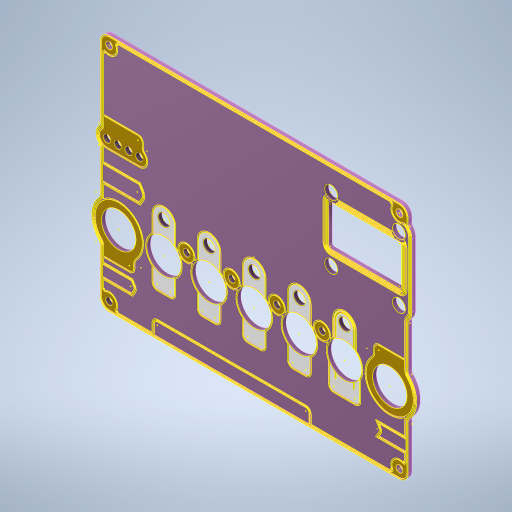
# Autodesk Inventor part: top_cover_template
Saved by Autodesk Inventor 2024 (Build 280153000, 153)
## iProperties
Created: 2023-11-30
Part Number: top_cover_template
Material: Generic
Document SubType Name: Modeling
Designer: Ishaan
Density: 1 g/cm^3
Appearance: Smooth - Purple
Author: Ishaan
Autodesk Inventor part; units mm, degrees
(part 1 of 4)
ref_plane "YZ Plane" through (0, 0, 0) normal (1, 0, 0) x (0, 1, 0)
ref_plane "XZ Plane" through (0, 0, 0) normal (0, 1, 0) x (-1, 0, 0)
ref_plane "XY Plane" through (0, 0, 0) normal (0, 0, 1) x (1, 0, 0)
sketch "Sketch1" plane through (0, 0, 0) normal (0, 0, 1) x (1, 0, 0)
  line L0 (71.5, -55.5) -> (-71.5, -55.5)
  line L1 (-71.5, -55.5) -> (-71.5, 55.5)
  line L2 (-71.5, 55.5) -> (71.5, 55.5)
  line L3 (71.5, 55.5) -> (71.5, -55.5)
  line L4 (71.5, -55.5) -> (-71.5, 55.5) construction
  line L5 (-71.5, -55.5) -> (71.5, 55.5) construction
  point P0 (0, 0)
  dimension "d0" = 143
  dimension "d1" = 111
  constraints: 12 end point, 2 midpoint, 2 parallel, 1 horizontal, 1 perpendicular
  measures "d0" distance of L1.end L2.end
  measures "d1" distance of L0.end L1.end
extrude "Extrusion1" add sketch "Sketch1" along normal blind 1.6
fillet "Fillet1" radius 4 4 edges at (71.5, 55.5, 0.8) (-71.5, 55.5, 0.8) (-71.5, -55.5, 0.8) (71.5, -55.5, 0.8)
sketch "Sketch2" plane through (0, 0, 1.6) normal (0, 0, 1) x (1, 0, 0)
  arc A0 (67.5, -55.5) -> (71.5, -51.5) centre (67.5, -51.5) ccw projected
  line L0 (71.5, -51.5) -> (71.5, 51.5) projected
  arc A1 (71.5, 51.5) -> (67.5, 55.5) centre (67.5, 51.5) ccw projected
  line L1 (67.5, 55.5) -> (-67.5, 55.5) projected
  arc A2 (-67.5, 55.5) -> (-71.5, 51.5) centre (-67.5, 51.5) ccw projected
  line L2 (-71.5, 51.5) -> (-71.5, -51.5) projected
  arc A3 (-71.5, -51.5) -> (-67.5, -55.5) centre (-67.5, -51.5) ccw projected
  line L3 (-67.5, -55.5) -> (67.5, -55.5) projected
  line L4 (-31.5, -14) -> (31.5, -14) construction
  line L5 (-10.5, -14) -> (10.5, -14) construction
  point P0 (0, 0)
  point P1 (0, -14)
  dimension "d9" = 21
  dimension "d17" = 21
  dimension "d18" = 41.5
  constraints: 8 coincident, 4 end point, 2 midpoint, 2 point on line, 1 horizontal, 1 vertical alignment
  measures "d9" distance of L5.start point (-31.5, -14)
  measures "d17" distance of point (10.5, -14) point (-10.5, -14)
  measures "d18" distance between parallel lines of L3 L4
hole "Hole1" at (-31.5, -14, 1.6) at (31.5, -14, 1.6) at (-10.5, -14, 1.6) at (10.5, -14, 1.6) at (-67.5, 51.5, 1.6) at (67.5, 51.5, 1.6) at (67.5, -51.5, 1.6) at (-67.5, -51.5, 1.6) direction (0, 0, -1) diameter 3.2 end through all
sketch "Sketch3" plane through (0, 0, 1.6) normal (0, 0, 1) x (1, 0, 0)
  line L0 (-67.5, -55.5) -> (67.5, -55.5) projected
  line L1 (-63, -20.5) -> (63, -20.5) construction
  point P0 (0, 0)
  point P1 (-42, -20.5)
  point P2 (-21, -20.5)
  point P3 (0, -20.5)
  point P4 (21, -20.5)
  point P5 (42, -20.5)
  dimension "d21" = 21
  dimension "d26" = 35
  constraints: 2 end point, 2 horizontal, 1 vertical alignment, 6 other
  measures "d21" distance of L1.start point (-42, -20.5)
  measures "d26" distance between parallel lines of L0 L1
hole "Hole2" at (-63, -20.5, 1.6) at (-42, -20.5, 1.6) at (-21, -20.5, 1.6) at (0, -20.5, 1.6) at (21, -20.5, 1.6) at (42, -20.5, 1.6) at (63, -20.5, 1.6) direction (0, 0, -1) diameter 16 end through all
sketch "Sketch4" plane through (0, 0, 1.6) normal (0, 0, 1) x (1, 0, 0)
  circle A0 centre (63, -20.5) radius 8 projected
  circle A1 centre (42, -20.5) radius 8 projected
  circle A2 centre (21, -20.5) radius 8 projected
  circle A3 centre (0, -20.5) radius 8 projected
  circle A4 centre (-21, -20.5) radius 8 projected
  circle A5 centre (-42, -20.5) radius 8 projected
  circle A6 centre (-63, -20.5) radius 8 projected
  circle A7 centre (-67.5, -51.5) radius 1.6 projected
  circle A8 centre (67.5, -51.5) radius 1.6 projected
  circle A9 centre (67.5, 51.5) radius 1.6 projected
  circle A10 centre (-67.5, 51.5) radius 1.6 projected
  circle A11 centre (10.5, -14) radius 1.6 projected
  circle A12 centre (-10.5, -14) radius 1.6 projected
  circle A13 centre (31.5, -14) radius 1.6 projected
  circle A14 centre (-31.5, -14) radius 1.6 projected
  arc A15 (67.5, -55.5) -> (71.5, -51.5) centre (67.5, -51.5) ccw projected
  line L0 (71.5, -51.5) -> (71.5, 51.5) projected
  arc A16 (71.5, 51.5) -> (67.5, 55.5) centre (67.5, 51.5) ccw projected
  line L1 (67.5, 55.5) -> (-67.5, 55.5) projected
  arc A17 (-67.5, 55.5) -> (-71.5, 51.5) centre (-67.5, 51.5) ccw projected
  line L2 (-71.5, 51.5) -> (-71.5, -51.5) projected
  arc A18 (-71.5, -51.5) -> (-67.5, -55.5) centre (-67.5, -51.5) ccw projected
  line L3 (-67.5, -55.5) -> (67.5, -55.5) projected
  line L4 (-63, -20.5) -> (63, -20.5) construction
  line L5 (-63, -33) -> (63, -33)
  line L6 (63, -8) -> (-63, -8)
  arc A19 (-63, -8) -> (-63, -33) centre (-63, -20.5) ccw
  arc A20 (63, -33) -> (63, -8) centre (63, -20.5) ccw
  point P0 (71.5, -11.3348)
  point P1 (71.5, -29.6652)
  point P2 (-71.5, -29.6652)
  point P3 (-71.5, -11.3348)
  dimension "d125" = 25
  constraints: 8 end point, 4 point on circle, 4 tangent, 2 centre point, 1 horizontal, 1 midpoint, 1 parallel
  measures "d125" distance between parallel lines of L5 L6
extrude "Extrusion11" add sketch "Sketch4" against normal up to surface (1.6 mm away) contours L0 A20 | A19 L2
fillet "Fillet2" radius 2 4 edges at (71.5, -29.6652, 0.8) (71.5, -11.3348, 0.8) (-71.5, -11.3348, 0.8) (-71.5, -29.6652, 0.8)
sketch "Sketch5" plane through (0, 0, 1.6) normal (0, 0, 1) x (1, 0, 0)
  line L0 (-42, -6) -> (42, -6) construction
  line L1 (-67.5, -55.5) -> (67.5, -55.5) projected
  circle A0 centre (-42, -20.5) radius 8 projected
  circle A1 centre (-21, -20.5) radius 8 projected
  circle A2 centre (0, -20.5) radius 8 projected
  circle A3 centre (21, -20.5) radius 8 projected
  circle A4 centre (42, -20.5) radius 8 projected
  point P0 (0, 0)
  point P1 (0, -6)
  point P2 (0, -55.5)
  point P3 (-21, -6)
  point P4 (0, -6)
  point P5 (21, -6)
  dimension "d39" = 49.5
  constraints: 7 vertical alignment, 3 midpoint, 3 point on line, 2 end point, 1 coincident, 1 horizontal
  measures "d39" distance between parallel lines of L1 L0
hole "Hole3" at (-42, -6, 1.6) at (-21, -6, 1.6) at (0, -6, 1.6) at (21, -6, 1.6) at (42, -6, 1.6) direction (0, 0, -1) diameter 5.5 end through all
sketch "Sketch6" plane through (0, 0, 1.6) normal (0, 0, 1) x (1, 0, 0)
  line L0 (-67.5, -55.5) -> (67.5, -55.5) construction
  line L1 (-71.5, 51.5) -> (-71.5, -10.5) construction
  point P0 (0, 0)
  point P1 (-68.5, 13.5)
  point P2 (-63.5, 13.5)
  point P3 (-58.5, 13.5)
  point P4 (-53.5, 13.5)
  point P5 (-71.5, -11.2624)
  dimension "d49" = 5
  dimension "d54" = 69
  dimension "d55" = 3
  constraints: 1 horizontal, 3 other
  measures "d49" distance of point (-68.5, 13.5) point (-63.5, 13.5)
  measures "d54" distance from line of point (-68.5, 13.5) L0
  measures "d55" distance from line of point (-68.5, 13.5) L1
hole "Hole4" at (-68.5, 13.5, 1.6) at (-63.5, 13.5, 1.6) at (-58.5, 13.5, 1.6) at (-53.5, 13.5, 1.6) direction (0, 0, -1) diameter 3.4 end through all
sketch "Sketch7" plane through (0, 0, 1.6) normal (0, 0, 1) x (1, 0, 0)
  line L0 (-71.5, 51.5) -> (-71.5, -10.5) projected
  line L1 (-68.5, 13.5) -> (-53.5, 13.5) construction
  line L2 (-68.5, 8.5) -> (-53.5, 8.5)
  line L3 (-53.5, 18.5) -> (-68.5, 18.5)
  arc A0 (-68.5, 18.5) -> (-68.5, 8.5) centre (-68.5, 13.5) ccw
  arc A1 (-53.5, 8.5) -> (-53.5, 18.5) centre (-53.5, 13.5) ccw
  circle A2 centre (-53.5, 13.5) radius 1.7 projected
  circle A3 centre (-68.5, 13.5) radius 1.7 projected
  point P0 (0, 0)
  point P1 (-71.5, -11.2624)
  point P2 (-61, 13.5)
  point P3 (-71.5, 9.5)
  point P4 (-71.5, 17.5)
  dimension "d128" = 10
  constraints: 8 end point, 4 point on circle, 4 tangent, 2 centre point, 2 coincident, 1 horizontal, 1 midpoint, 1 parallel
  measures "d128" distance between parallel lines of L2 L3
extrude "Extrusion3" add sketch "Sketch7" against normal up to surface (1.6 mm away) contours L0 A0
fillet "Fillet3" radius 0.75 2 edges at (-71.5, 9.5, 0.8) (-71.5, 17.5, 0.8)
sketch "Sketch8" plane through (0, 0, 1.6) normal (0, 0, 1) x (1, 0, 0)
  line L0 (68.5, 21.1) -> (34.5, 21.1)
  line L1 (34.5, 21.1) -> (34.5, 40.1)
  line L2 (34.5, 40.1) -> (68.5, 40.1)
  line L3 (68.5, 40.1) -> (68.5, 21.1)
  line L4 (68.5, 21.1) -> (34.5, 40.1) construction
  line L5 (34.5, 21.1) -> (68.5, 40.1) construction
  line L6 (71.5, -10.5) -> (71.5, 51.5) projected
  line L7 (-67.5, -55.5) -> (67.5, -55.5) projected
  point P0 (0, 0)
  point P1 (51.5, 30.6)
  point P2 (71.5, -11.2624)
  dimension "d67" = 20
  dimension "d68" = 86.1
  dimension "d69" = 34
  dimension "d70" = 19
  constraints: 12 end point, 2 midpoint, 2 parallel, 1 horizontal, 1 perpendicular
  measures "d67" distance from line of L6 point (51.5, 30.6)
  measures "d68" distance from line of L7 point (51.5, 30.6)
  measures "d69" distance of L1.end L2.end
  measures "d70" distance of L2.end L0.start
extrude "Extrusion4" cut sketch "Sketch8" against normal through all
fillet "Fillet4" radius 1 4 edges at (34.5, 40.1, 0.8) (34.5, 21.1, 0.8) (68.5, 40.1, 0.8) (68.5, 21.1, 0.8)
sketch "Sketch9" plane through (0, 0, 1.6) normal (0, 0, 1) x (1, 0, 0)
  line L0 (67.25, 14.25) -> (35.75, 14.25)
  line L1 (35.75, 14.25) -> (35.75, 43.95)
  line L2 (35.75, 43.95) -> (67.25, 43.95)
  line L3 (67.25, 43.95) -> (67.25, 14.25)
  line L4 (67.25, 14.25) -> (35.75, 43.95) construction
  line L5 (35.75, 14.25) -> (67.25, 43.95) construction
  line L6 (-67.5, -55.5) -> (67.5, -55.5) projected
  point P0 (0, 0)
  point P1 (51.5, 29.1)
  point P2 (51.5, 30.6)
  dimension "d74" = 31.5
  dimension "d75" = 29.7
  dimension "d76" = 69.75
  constraints: 12 end point, 4 coincident, 2 midpoint, 2 parallel, 1 horizontal, 1 perpendicular, 1 vertical alignment
  measures "d74" distance of L1.end L2.end
  measures "d75" distance of L2.end L0.start
  measures "d76" distance between parallel lines of L6 L0
hole "Hole5" at (51.5, 30.6, 1.6) at (35.75, 43.95, 1.6) at (67.25, 43.95, 1.6) at (67.25, 14.25, 1.6) at (35.75, 14.25, 1.6) direction (0, 0, -1) diameter 6 end through all
sketch "Sketch10" plane through (0, 0, 1.6) normal (0, 0, 1) x (1, 0, 0)
  circle A0 centre (35.75, 14.25) radius 3 projected
  circle A1 centre (67.25, 14.25) radius 3 projected
  circle A2 centre (67.25, 43.95) radius 3 projected
  circle A3 centre (35.75, 43.95) radius 3 projected
  line L0 (34.5, 22.1) -> (34.5, 39.1) projected
  arc A4 (35.5, 40.1) -> (34.5, 39.1) centre (35.5, 39.1) ccw projected
  line L1 (35.5, 40.1) -> (67.5, 40.1) projected
  arc A5 (68.5, 39.1) -> (67.5, 40.1) centre (67.5, 39.1) ccw projected
  line L2 (68.5, 39.1) -> (68.5, 22.1) projected
  arc A6 (67.5, 21.1) -> (68.5, 22.1) centre (67.5, 22.1) ccw projected
  line L3 (67.5, 21.1) -> (35.5, 21.1) projected
  arc A7 (34.5, 22.1) -> (35.5, 21.1) centre (35.5, 22.1) ccw projected
  circle A8 centre (-53.5, 13.5) radius 1.7 projected
  circle A9 centre (-58.5, 13.5) radius 1.7 projected
  circle A10 centre (-63.5, 13.5) radius 1.7 projected
  circle A11 centre (-68.5, 13.5) radius 1.7 projected
  circle A12 centre (42, -6) radius 2.75 projected
  circle A13 centre (21, -6) radius 2.75 projected
  circle A14 centre (0, -6) radius 2.75 projected
  circle A15 centre (-21, -6) radius 2.75 projected
  circle A16 centre (-42, -6) radius 2.75 projected
  circle A17 centre (63, -20.5) radius 8 projected
  circle A18 centre (42, -20.5) radius 8 projected
  circle A19 centre (21, -20.5) radius 8 projected
  circle A20 centre (0, -20.5) radius 8 projected
  circle A21 centre (-21, -20.5) radius 8 projected
  circle A22 centre (-42, -20.5) radius 8 projected
  circle A23 centre (-63, -20.5) radius 8 projected
  circle A24 centre (-67.5, -51.5) radius 1.6 projected
  circle A25 centre (67.5, -51.5) radius 1.6 projected
  circle A26 centre (67.5, 51.5) radius 1.6 projected
  circle A27 centre (-67.5, 51.5) radius 1.6 projected
  circle A28 centre (10.5, -14) radius 1.6 projected
  circle A29 centre (-10.5, -14) radius 1.6 projected
  circle A30 centre (31.5, -14) radius 1.6 projected
  circle A31 centre (-31.5, -14) radius 1.6 projected
  line L4 (-71.5, 9.1411) -> (-71.5, -10.5) projected
  line L5 (-71.5, -30.5) -> (-71.5, -51.5) projected
  arc A32 (-71.5, -51.5) -> (-67.5, -55.5) centre (-67.5, -51.5) ccw projected
  line L6 (-67.5, -55.5) -> (67.5, -55.5) projected
  arc A33 (67.5, -55.5) -> (71.5, -51.5) centre (67.5, -51.5) ccw projected
  line L7 (71.5, -51.5) -> (71.5, -30.5) projected
  line L8 (71.5, -10.5) -> (71.5, 51.5) projected
  arc A34 (71.5, 51.5) -> (67.5, 55.5) centre (67.5, 51.5) ccw projected
  line L9 (67.5, 55.5) -> (-67.5, 55.5) projected
  arc A35 (-67.5, 55.5) -> (-71.5, 51.5) centre (-67.5, 51.5) ccw projected
  line L10 (-71.5, 51.5) -> (-71.5, 17.8589) projected
  arc A36 (72.0517, -29.1207) -> (71.5, -30.5) centre (73.5, -30.5) ccw projected
  arc A37 (72.0517, -29.1207) -> (72.0517, -11.8793) centre (63, -20.5) ccw projected
  arc A38 (71.5, -10.5) -> (72.0517, -11.8793) centre (73.5, -10.5) ccw projected
  arc A39 (-71.7609, 17.2903) -> (-71.5, 17.8589) centre (-72.25, 17.8589) ccw projected
  arc A40 (-71.7609, 17.2903) -> (-71.7609, 9.7097) centre (-68.5, 13.5) ccw projected
  arc A41 (-71.5, 9.1411) -> (-71.7609, 9.7097) centre (-72.25, 9.1411) ccw projected
  arc A42 (-72.0517, -11.8793) -> (-71.5, -10.5) centre (-73.5, -10.5) ccw projected
  arc A43 (-72.0517, -11.8793) -> (-72.0517, -29.1207) centre (-63, -20.5) ccw projected
  arc A44 (-71.5, -30.5) -> (-72.0517, -29.1207) centre (-73.5, -30.5) ccw projected
  line L11 (67.25, 43.95) -> (67.25, 14.25) construction
  line L12 (61.25, 43.95) -> (61.25, 14.25)
  line L13 (73.25, 14.25) -> (73.25, 43.95)
  arc A45 (73.25, 43.95) -> (61.25, 43.95) centre (67.25, 43.95) ccw
  arc A46 (61.25, 14.25) -> (73.25, 14.25) centre (67.25, 14.25) ccw
  point P0 (0, 0)
  point P1 (67.25, 29.1)
  point P2 (71.5, 48.1853)
  point P3 (71.5, 10.0147)
  dimension "d129" = 12
  constraints: 8 end point, 4 point on circle, 4 tangent, 2 centre point, 1 midpoint, 1 parallel, 1 vertical
  measures "d129" distance between parallel lines of L13 L12
extrude "Extrusion5" add sketch "Sketch10" against normal up to surface (1.6 mm away) contours L8 A45 L13 A46
fillet "Fillet5" radius 1 2 edges at (71.5, 10.0147, 0.8) (71.5, 48.1853, 0.8)
sketch "Sketch11" plane through (0, 0, 1.6) normal (0, 0, 1) x (1, 0, 0)
  circle A0 centre (35.75, 14.25) radius 3 construction
  circle A1 centre (67.25, 14.25) radius 3 construction
  circle A2 centre (67.25, 43.95) radius 3 construction
  circle A3 centre (35.75, 43.95) radius 3 construction
  line L0 (34.5, 22.1) -> (34.5, 39.1) construction
  arc A4 (35.5, 40.1) -> (34.5, 39.1) centre (35.5, 39.1) ccw construction
  line L1 (35.5, 40.1) -> (67.5, 40.1) construction
  arc A5 (68.5, 39.1) -> (67.5, 40.1) centre (67.5, 39.1) ccw construction
  line L2 (68.5, 39.1) -> (68.5, 22.1) construction
  arc A6 (67.5, 21.1) -> (68.5, 22.1) centre (67.5, 22.1) ccw construction
  line L3 (67.5, 21.1) -> (35.5, 21.1) construction
  arc A7 (34.5, 22.1) -> (35.5, 21.1) centre (35.5, 22.1) ccw construction
  circle A8 centre (-53.5, 13.5) radius 1.7 construction
  circle A9 centre (-58.5, 13.5) radius 1.7 construction
  circle A10 centre (-63.5, 13.5) radius 1.7 construction
  circle A11 centre (-68.5, 13.5) radius 1.7 construction
  circle A12 centre (42, -6) radius 2.75 construction
  circle A13 centre (21, -6) radius 2.75 construction
  circle A14 centre (0, -6) radius 2.75 construction
  circle A15 centre (-21, -6) radius 2.75 construction
  circle A16 centre (-42, -6) radius 2.75 construction
  circle A17 centre (63, -20.5) radius 8 construction
  circle A18 centre (42, -20.5) radius 8 construction
  circle A19 centre (21, -20.5) radius 8 construction
  circle A20 centre (0, -20.5) radius 8 construction
  circle A21 centre (-21, -20.5) radius 8 construction
  circle A22 centre (-42, -20.5) radius 8 construction
  circle A23 centre (-63, -20.5) radius 8 construction
  circle A24 centre (-67.5, -51.5) radius 1.6 projected
  circle A25 centre (67.5, -51.5) radius 1.6 projected
  circle A26 centre (67.5, 51.5) radius 1.6 projected
  circle A27 centre (-67.5, 51.5) radius 1.6 projected
  circle A28 centre (10.5, -14) radius 1.6 projected
  circle A29 centre (-10.5, -14) radius 1.6 projected
  circle A30 centre (31.5, -14) radius 1.6 projected
  circle A31 centre (-31.5, -14) radius 1.6 projected
  line L4 (71.5, 48.5801) -> (71.5, 51.5) projected
  arc A32 (71.5, 51.5) -> (67.5, 55.5) centre (67.5, 51.5) ccw projected
  line L5 (67.5, 55.5) -> (-67.5, 55.5) projected
  arc A33 (-67.5, 55.5) -> (-71.5, 51.5) centre (-67.5, 51.5) ccw projected
  line L6 (-71.5, 51.5) -> (-71.5, 17.8589) projected
  line L7 (-71.5, 9.1411) -> (-71.5, -10.5) projected
  line L8 (-71.5, -30.5) -> (-71.5, -51.5) projected
  arc A34 (-71.5, -51.5) -> (-67.5, -55.5) centre (-67.5, -51.5) ccw projected
  line L9 (-67.5, -55.5) -> (67.5, -55.5) projected
  arc A35 (67.5, -55.5) -> (71.5, -51.5) centre (67.5, -51.5) ccw projected
  line L10 (71.5, -51.5) -> (71.5, -30.5) projected
  line L11 (71.5, -10.5) -> (71.5, 9.6199) projected
  arc A36 (72.0517, -29.1207) -> (71.5, -30.5) centre (73.5, -30.5) ccw projected
  arc A37 (72.0517, -29.1207) -> (72.0517, -11.8793) centre (63, -20.5) ccw projected
  arc A38 (71.5, -10.5) -> (72.0517, -11.8793) centre (73.5, -10.5) ccw projected
  arc A39 (71.75, 10.2814) -> (71.5, 9.6199) centre (72.5, 9.6199) ccw projected
  arc A40 (71.75, 10.2814) -> (73.25, 14.25) centre (67.25, 14.25) ccw projected
  line L12 (73.25, 14.25) -> (73.25, 43.95) projected
  arc A41 (73.25, 43.95) -> (71.75, 47.9186) centre (67.25, 43.95) ccw projected
  arc A42 (71.5, 48.5801) -> (71.75, 47.9186) centre (72.5, 48.5801) ccw projected
  arc A43 (-71.7609, 17.2903) -> (-71.5, 17.8589) centre (-72.25, 17.8589) ccw projected
  arc A44 (-71.7609, 17.2903) -> (-71.7609, 9.7097) centre (-68.5, 13.5) ccw projected
  arc A45 (-71.5, 9.1411) -> (-71.7609, 9.7097) centre (-72.25, 9.1411) ccw projected
  arc A46 (-72.0517, -11.8793) -> (-71.5, -10.5) centre (-73.5, -10.5) ccw projected
  arc A47 (-72.0517, -11.8793) -> (-72.0517, -29.1207) centre (-63, -20.5) ccw projected
  arc A48 (-71.5, -30.5) -> (-72.0517, -29.1207) centre (-73.5, -30.5) ccw projected
  arc A49 (-67.5, 55) -> (-71, 51.5) centre (-67.5, 51.5) ccw
  line L13 (-67.5, 55) -> (67.5, 55)
  arc A50 (71, 51.5) -> (67.5, 55) centre (67.5, 51.5) ccw
  line L14 (71, 51.5) -> (71, 48.5801)
  arc A51 (71, 48.5801) -> (71.375, 47.5879) centre (72.5, 48.5801) ccw
  arc A52 (72.75, 43.95) -> (71.375, 47.5879) centre (67.25, 43.95) ccw
  line L15 (72.75, 43.95) -> (72.75, 14.25)
  arc A53 (71.375, 10.6121) -> (72.75, 14.25) centre (67.25, 14.25) ccw
  arc A54 (71.375, 10.6121) -> (71, 9.6199) centre (72.5, 9.6199) ccw
  line L16 (71, 9.6199) -> (71, -10.5)
  arc A55 (71, -10.5) -> (71.6897, -12.2241) centre (73.5, -10.5) ccw
  arc A56 (71.6897, -28.7759) -> (71.6897, -12.2241) centre (63, -20.5) ccw
  arc A57 (71.6897, -28.7759) -> (71, -30.5) centre (73.5, -30.5) ccw
  line L17 (71, -30.5) -> (71, -51.5)
  arc A58 (67.5, -55) -> (71, -51.5) centre (67.5, -51.5) ccw
  line L18 (67.5, -55) -> (-67.5, -55)
  arc A59 (-71, -51.5) -> (-67.5, -55) centre (-67.5, -51.5) ccw
  line L19 (-71, -51.5) -> (-71, -30.5)
  arc A60 (-71, -30.5) -> (-71.6897, -28.7759) centre (-73.5, -30.5) ccw
  arc A61 (-71.6897, -12.2241) -> (-71.6897, -28.7759) centre (-63, -20.5) ccw
  arc A62 (-71.6897, -12.2241) -> (-71, -10.5) centre (-73.5, -10.5) ccw
  line L20 (-71, -10.5) -> (-71, 9.1411)
  arc A63 (-71, 9.1411) -> (-71.4348, 10.0887) centre (-72.25, 9.1411) ccw
  arc A64 (-71.4348, 16.9113) -> (-71.4348, 10.0887) centre (-68.5, 13.5) ccw
  arc A65 (-71.4348, 16.9113) -> (-71, 17.8589) centre (-72.25, 17.8589) ccw
  line L21 (-71, 17.8589) -> (-71, 51.5)
  arc A66 (-67.5, 54.5) -> (-70.5, 51.5) centre (-67.5, 51.5) ccw
  line L22 (-67.5, 54.5) -> (67.5, 54.5)
  arc A67 (70.5, 51.5) -> (67.5, 54.5) centre (67.5, 51.5) ccw
  line L23 (70.5, 51.5) -> (70.5, 48.5801)
  arc A68 (70.5, 48.5801) -> (71, 47.2572) centre (72.5, 48.5801) ccw
  arc A69 (72.25, 43.95) -> (71, 47.2572) centre (67.25, 43.95) ccw
  line L24 (72.25, 43.95) -> (72.25, 14.25)
  arc A70 (71, 10.9428) -> (72.25, 14.25) centre (67.25, 14.25) ccw
  arc A71 (71, 10.9428) -> (70.5, 9.6199) centre (72.5, 9.6199) ccw
  line L25 (70.5, 9.6199) -> (70.5, -10.5)
  arc A72 (70.5, -10.5) -> (71.3276, -12.569) centre (73.5, -10.5) ccw
  arc A73 (71.3276, -28.431) -> (71.3276, -12.569) centre (63, -20.5) ccw
  arc A74 (71.3276, -28.431) -> (70.5, -30.5) centre (73.5, -30.5) ccw
  line L26 (70.5, -30.5) -> (70.5, -51.5)
  arc A75 (67.5, -54.5) -> (70.5, -51.5) centre (67.5, -51.5) ccw
  line L27 (67.5, -54.5) -> (-67.5, -54.5)
  arc A76 (-70.5, -51.5) -> (-67.5, -54.5) centre (-67.5, -51.5) ccw
  line L28 (-70.5, -51.5) -> (-70.5, -30.5)
  arc A77 (-70.5, -30.5) -> (-71.3276, -28.431) centre (-73.5, -30.5) ccw
  arc A78 (-71.3276, -12.569) -> (-71.3276, -28.431) centre (-63, -20.5) ccw
  arc A79 (-71.3276, -12.569) -> (-70.5, -10.5) centre (-73.5, -10.5) ccw
  line L29 (-70.5, -10.5) -> (-70.5, 9.1411)
  arc A80 (-70.5, 9.1411) -> (-71.1087, 10.4677) centre (-72.25, 9.1411) ccw
  arc A81 (-71.1087, 16.5323) -> (-71.1087, 10.4677) centre (-68.5, 13.5) ccw
  arc A82 (-71.1087, 16.5323) -> (-70.5, 17.8589) centre (-72.25, 17.8589) ccw
  line L30 (-70.5, 17.8589) -> (-70.5, 51.5)
  circle A83 centre (67.5, -51.5) radius 3.5
  circle A84 centre (-67.5, -51.5) radius 3.5
  circle A85 centre (-31.5, -14) radius 3.5
  circle A86 centre (-10.5, -14) radius 3.5
  circle A87 centre (10.5, -14) radius 3.5
  circle A88 centre (31.5, -14) radius 3.5
  circle A89 centre (67.5, 51.5) radius 3.5
  circle A90 centre (-67.5, 51.5) radius 3.5
  point P0 (-70.5, 49.6972)
  point P1 (-65.6972, 54.5)
  point P2 (65.6972, 54.5)
  point P3 (70.5, 49.6972)
  point P4 (70.5, -49.6972)
  point P5 (65.6972, -54.5)
  point P6 (-65.6972, -54.5)
  point P7 (-70.5, -49.6972)
  dimension "d130" = 0.5
  dimension "d131" = 0.5
  dimension "d132" = 7
  constraints: 68 point on circle, 42 centre point, 36 end point, 8 coincident, 7 equal radius, 50 other
  measures "d130" radial gap between concentric circles of A33 A49
  measures "d131" radial gap between concentric circles of A49 A66
  measures "d132" diameter of A83
extrude "Extrusion6" add sketch "Sketch11" along normal blind 0.01 contours A90 L22 A66 L30 A49 | L13 A89 L22 A90 | A90 L30 A82 A81 A80 L29 A79 A78 A77 L28 A84 L19 A60 A61 A62 L20 A63 A64 A65 L21 | A50 A89 L23 A67 L22 | A90 L30 A66 L22 | L14 A51 A52 L15 A53 A54 L16 A55 A56 A57 L17 A83 L26 A74 A73 A72 L25 A71 A70 L24 A69 A68 L23 A89 | L22 A67 L23 A89 | A84 L28 A76 L27 A59 | A84 L27 A83 L18 | A84 L27 A76 L28 | A83 L27 A75 L26 A58 | A83 L26 A75 L27 | A85 | A86 | A87 | A88
fillet "Fillet6" radius 1 8 edges at (65.6972, 54.5, 1.605) (70.5, 49.6972, 1.605) (-70.5, 49.6972, 1.605) (-65.6972, 54.5, 1.605) (-70.5, -49.6972, 1.605) (-65.6972, -54.5, 1.605) (70.5, -49.6972, 1.605) (65.6972, -54.5, 1.605)
sketch "Sketch12" plane through (0, 0, 1.6) normal (0, 0, 1) x (1, 0, 0)
  circle A0 centre (-63, -20.5) radius 8 projected
  circle A1 centre (-42, -20.5) radius 8 projected
  circle A2 centre (-21, -20.5) radius 8 projected
  circle A3 centre (0, -20.5) radius 8 projected
  circle A4 centre (21, -20.5) radius 8 projected
  circle A5 centre (42, -20.5) radius 8 projected
  circle A6 centre (63, -20.5) radius 8 projected
  circle A7 centre (-42, -6) radius 2.75 projected
  circle A8 centre (-21, -6) radius 2.75 projected
  circle A9 centre (0, -6) radius 2.75 projected
  circle A10 centre (21, -6) radius 2.75 projected
  circle A11 centre (42, -6) radius 2.75 projected
  circle A12 centre (-68.5, 13.5) radius 1.7 projected
  circle A13 centre (-63.5, 13.5) radius 1.7 projected
  circle A14 centre (-58.5, 13.5) radius 1.7 projected
  circle A15 centre (-53.5, 13.5) radius 1.7 projected
  line L0 (34.5, 22.1) -> (34.5, 39.1) projected
  arc A16 (35.5, 40.1) -> (34.5, 39.1) centre (35.5, 39.1) ccw projected
  line L1 (35.5, 40.1) -> (67.5, 40.1) projected
  arc A17 (68.5, 39.1) -> (67.5, 40.1) centre (67.5, 39.1) ccw projected
  line L2 (68.5, 39.1) -> (68.5, 22.1) projected
  arc A18 (67.5, 21.1) -> (68.5, 22.1) centre (67.5, 22.1) ccw projected
  line L3 (67.5, 21.1) -> (35.5, 21.1) projected
  arc A19 (34.5, 22.1) -> (35.5, 21.1) centre (35.5, 22.1) ccw projected
  circle A20 centre (35.75, 43.95) radius 3 projected
  circle A21 centre (67.25, 43.95) radius 3 projected
  circle A22 centre (67.25, 14.25) radius 3 projected
  circle A23 centre (35.75, 14.25) radius 3 projected
  line L4 (-42, -6) -> (-42, -20.5) construction
  line L5 (-47, -6) -> (-47, -20.5)
  line L6 (-37, -20.5) -> (-37, -6)
  arc A24 (-37, -6) -> (-47, -6) centre (-42, -6) ccw
  arc A25 (-47, -20.5) -> (-37, -20.5) centre (-42, -20.5) ccw
  line L7 (-47, -26.745) -> (-37, -26.745)
  line L8 (-37, -26.745) -> (-37, -33.5)
  line L9 (-39, -35.5) -> (-45, -35.5)
  line L10 (-47, -33.5) -> (-47, -26.745)
  arc A26 (-47, -33.5) -> (-45, -35.5) centre (-45, -33.5) ccw
  arc A27 (-39, -35.5) -> (-37, -33.5) centre (-39, -33.5) ccw
  point P0 (0, 0)
  point P1 (-42, -13.25)
  point P2 (-42, -26.745)
  point P3 (-47, -14.255)
  point P4 (-37, -14.255)
  dimension "d95" = 10
  dimension "d98" = 7
  dimension "d100" = 2
  constraints: 16 end point, 10 point on circle, 8 tangent, 4 centre point, 3 parallel, 2 midpoint, 1 coincident, 1 collinear, 1 equal radius, 1 horizontal, 1 perpendicular, 1 vertical, 1 vertical alignment
  measures "d95" diameter of A25
  measures "d98" distance edge to line of A1 L9
  measures "d100" radius of A26
extrude "Extrusion7" add sketch "Sketch12" along normal blind 0.005 contours A1 L8 A27 L9 A26 L10 | L5 A24 L6 A1
pattern_linear "Rectangular Pattern1" count 4 spacing 21 along (1, 0, 0) of "Extrusion7"
sketch "Sketch13" plane through (0, 0, 1.6) normal (0, 0, 1) x (1, 0, 0)
  line L0 (16, -33.5) -> (16, -26.745) projected
  arc A0 (16, -14.255) -> (16, -26.745) centre (21, -20.5) ccw projected
  line L1 (16, -14.255) -> (16, -6) projected
  arc A1 (26, -6) -> (16, -6) centre (21, -6) ccw projected
  line L2 (26, -6) -> (26, -14.255) projected
  arc A2 (26, -26.745) -> (26, -14.255) centre (21, -20.5) ccw projected
  line L3 (26, -26.745) -> (26, -33.5) projected
  arc A3 (24, -35.5) -> (26, -33.5) centre (24, -33.5) ccw projected
  line L4 (24, -35.5) -> (18, -35.5) projected
  arc A4 (16, -33.5) -> (18, -35.5) centre (18, -33.5) ccw projected
  line L5 (-5, -33.5) -> (-5, -26.745) projected
  arc A5 (-5, -14.255) -> (-5, -26.745) centre (0, -20.5) ccw projected
  line L6 (-5, -14.255) -> (-5, -6) projected
  arc A6 (5, -6) -> (-5, -6) centre (0, -6) ccw projected
  line L7 (5, -6) -> (5, -14.255) projected
  arc A7 (5, -26.745) -> (5, -14.255) centre (0, -20.5) ccw projected
  line L8 (5, -26.745) -> (5, -33.5) projected
  arc A8 (3, -35.5) -> (5, -33.5) centre (3, -33.5) ccw projected
  line L9 (3, -35.5) -> (-3, -35.5) projected
  arc A9 (-5, -33.5) -> (-3, -35.5) centre (-3, -33.5) ccw projected
  line L10 (-26, -33.5) -> (-26, -26.745) projected
  arc A10 (-26, -14.255) -> (-26, -26.745) centre (-21, -20.5) ccw projected
  line L11 (-26, -14.255) -> (-26, -6) projected
  arc A11 (-16, -6) -> (-26, -6) centre (-21, -6) ccw projected
  line L12 (-16, -6) -> (-16, -14.255) projected
  arc A12 (-16, -26.745) -> (-16, -14.255) centre (-21, -20.5) ccw projected
  line L13 (-16, -26.745) -> (-16, -33.5) projected
  arc A13 (-18, -35.5) -> (-16, -33.5) centre (-18, -33.5) ccw projected
  line L14 (-18, -35.5) -> (-24, -35.5) projected
  arc A14 (-26, -33.5) -> (-24, -35.5) centre (-24, -33.5) ccw projected
  line L15 (-47, -33.5) -> (-47, -26.745) projected
  arc A15 (-47, -14.255) -> (-47, -26.745) centre (-42, -20.5) ccw projected
  line L16 (-47, -14.255) -> (-47, -6) projected
  arc A16 (-37, -6) -> (-47, -6) centre (-42, -6) ccw projected
  line L17 (-37, -6) -> (-37, -14.255) projected
  arc A17 (-37, -26.745) -> (-37, -14.255) centre (-42, -20.5) ccw projected
  line L18 (-37, -26.745) -> (-37, -33.5) projected
  arc A18 (-39, -35.5) -> (-37, -33.5) centre (-39, -33.5) ccw projected
  line L19 (-39, -35.5) -> (-45, -35.5) projected
  arc A19 (-47, -33.5) -> (-45, -35.5) centre (-45, -33.5) ccw projected
  circle A20 centre (-63, -20.5) radius 8 projected
  circle A21 centre (42, -20.5) radius 8 projected
  circle A22 centre (63, -20.5) radius 8 projected
  circle A23 centre (42, -6) radius 2.75 projected
  circle A24 centre (-68.5, 13.5) radius 1.7 projected
  circle A25 centre (-63.5, 13.5) radius 1.7 projected
  circle A26 centre (-58.5, 13.5) radius 1.7 projected
  circle A27 centre (-53.5, 13.5) radius 1.7 projected
  line L20 (34.5, 22.1) -> (34.5, 39.1) projected
  arc A28 (35.5, 40.1) -> (34.5, 39.1) centre (35.5, 39.1) ccw projected
  line L21 (35.5, 40.1) -> (67.5, 40.1) projected
  arc A29 (68.5, 39.1) -> (67.5, 40.1) centre (67.5, 39.1) ccw projected
  line L22 (68.5, 39.1) -> (68.5, 22.1) projected
  arc A30 (67.5, 21.1) -> (68.5, 22.1) centre (67.5, 22.1) ccw projected
  line L23 (67.5, 21.1) -> (35.5, 21.1) projected
  arc A31 (34.5, 22.1) -> (35.5, 21.1) centre (35.5, 22.1) ccw projected
  circle A32 centre (35.75, 43.95) radius 3 projected
  circle A33 centre (67.25, 43.95) radius 3 projected
  circle A34 centre (67.25, 14.25) radius 3 projected
  circle A35 centre (35.75, 14.25) radius 3 projected
  line L24 (42, -6) -> (42, -20.5) construction
  line L25 (37, -6) -> (37, -20.5)
  line L26 (47, -20.5) -> (47, -6)
  arc A36 (47, -6) -> (37, -6) centre (42, -6) ccw
  arc A37 (37, -20.5) -> (47, -20.5) centre (42, -20.5) ccw
  arc A38 (26, -6) -> (16, -6) centre (21, -6) ccw projected
  line L27 (35, -24.373) -> (49, -24.373)
  line L28 (49, -24.373) -> (49, -33.5)
  line L29 (47, -35.5) -> (37, -35.5)
  line L30 (35, -33.5) -> (35, -24.373)
  line L31 (18, -35.5) -> (24, -35.5) projected
  arc A39 (35, -33.5) -> (37, -35.5) centre (37, -33.5) ccw
  arc A40 (47, -35.5) -> (49, -33.5) centre (47, -33.5) ccw
  arc A41 (24, -35.5) -> (26, -33.5) centre (24, -33.5) ccw projected
  point P0 (0, 0)
  point P1 (42, -13.25)
  point P2 (37, -14.255)
  point P3 (47, -14.255)
  dimension "d109" = 14
  constraints: 16 end point, 10 point on circle, 8 tangent, 4 centre point, 3 equal radius, 3 parallel, 1 collinear, 1 horizontal, 1 midpoint, 1 perpendicular, 1 vertical
  measures "d109" distance of L27.start L27.end
extrude "Extrusion8" add sketch "Sketch13" along normal up to surface (0.005 mm away) contours A21 L28 A40 L29 A39 L30 | L25 A36 L26 A21
sketch "Sketch14" plane through (0, 0, 1.6) normal (0, 0, 1) x (1, 0, 0)
  line L0 (35, -33.5) -> (35, -24.373) projected
  arc A0 (37, -14.255) -> (35, -24.373) centre (42, -20.5) ccw projected
  line L1 (37, -14.255) -> (37, -6) projected
  arc A1 (47, -6) -> (37, -6) centre (42, -6) ccw projected
  line L2 (47, -6) -> (47, -14.255) projected
  arc A2 (49, -24.373) -> (47, -14.255) centre (42, -20.5) ccw projected
  line L3 (49, -24.373) -> (49, -33.5) projected
  arc A3 (47, -35.5) -> (49, -33.5) centre (47, -33.5) ccw projected
  line L4 (47, -35.5) -> (37, -35.5) projected
  arc A4 (35, -33.5) -> (37, -35.5) centre (37, -33.5) ccw projected
  line L5 (16, -33.5) -> (16, -26.745) projected
  arc A5 (16, -14.255) -> (16, -26.745) centre (21, -20.5) ccw projected
  line L6 (16, -14.255) -> (16, -6) projected
  arc A6 (26, -6) -> (16, -6) centre (21, -6) ccw projected
  line L7 (26, -6) -> (26, -14.255) projected
  arc A7 (26, -26.745) -> (26, -14.255) centre (21, -20.5) ccw projected
  line L8 (26, -26.745) -> (26, -33.5) projected
  arc A8 (24, -35.5) -> (26, -33.5) centre (24, -33.5) ccw projected
  line L9 (24, -35.5) -> (18, -35.5) projected
  arc A9 (16, -33.5) -> (18, -35.5) centre (18, -33.5) ccw projected
  line L10 (-5, -33.5) -> (-5, -26.745) projected
  arc A10 (-5, -14.255) -> (-5, -26.745) centre (0, -20.5) ccw projected
  line L11 (-5, -14.255) -> (-5, -6) projected
  arc A11 (5, -6) -> (-5, -6) centre (0, -6) ccw projected
  line L12 (5, -6) -> (5, -14.255) projected
  arc A12 (5, -26.745) -> (5, -14.255) centre (0, -20.5) ccw projected
  line L13 (5, -26.745) -> (5, -33.5) projected
  arc A13 (3, -35.5) -> (5, -33.5) centre (3, -33.5) ccw projected
  line L14 (3, -35.5) -> (-3, -35.5) projected
  arc A14 (-5, -33.5) -> (-3, -35.5) centre (-3, -33.5) ccw projected
  line L15 (-26, -33.5) -> (-26, -26.745) projected
  arc A15 (-26, -14.255) -> (-26, -26.745) centre (-21, -20.5) ccw projected
  line L16 (-26, -14.255) -> (-26, -6) projected
  arc A16 (-16, -6) -> (-26, -6) centre (-21, -6) ccw projected
  line L17 (-16, -6) -> (-16, -14.255) projected
  arc A17 (-16, -26.745) -> (-16, -14.255) centre (-21, -20.5) ccw projected
  line L18 (-16, -26.745) -> (-16, -33.5) projected
  arc A18 (-18, -35.5) -> (-16, -33.5) centre (-18, -33.5) ccw projected
  line L19 (-18, -35.5) -> (-24, -35.5) projected
  arc A19 (-26, -33.5) -> (-24, -35.5) centre (-24, -33.5) ccw projected
  line L20 (-47, -33.5) -> (-47, -26.745) projected
  arc A20 (-47, -14.255) -> (-47, -26.745) centre (-42, -20.5) ccw projected
  line L21 (-47, -14.255) -> (-47, -6) projected
  arc A21 (-37, -6) -> (-47, -6) centre (-42, -6) ccw projected
  line L22 (-37, -6) -> (-37, -14.255) projected
  arc A22 (-37, -26.745) -> (-37, -14.255) centre (-42, -20.5) ccw projected
  line L23 (-37, -26.745) -> (-37, -33.5) projected
  arc A23 (-39, -35.5) -> (-37, -33.5) centre (-39, -33.5) ccw projected
  line L24 (-39, -35.5) -> (-45, -35.5) projected
  arc A24 (-47, -33.5) -> (-45, -35.5) centre (-45, -33.5) ccw projected
  circle A25 centre (-63, -20.5) radius 8 projected
  circle A26 centre (63, -20.5) radius 8 projected
  circle A27 centre (-68.5, 13.5) radius 1.7 projected
  circle A28 centre (-63.5, 13.5) radius 1.7 projected
  circle A29 centre (-58.5, 13.5) radius 1.7 projected
  circle A30 centre (-53.5, 13.5) radius 1.7 projected
  line L25 (34.5, 22.1) -> (34.5, 39.1) projected
  arc A31 (35.5, 40.1) -> (34.5, 39.1) centre (35.5, 39.1) ccw projected
  line L26 (35.5, 40.1) -> (67.5, 40.1) projected
  arc A32 (68.5, 39.1) -> (67.5, 40.1) centre (67.5, 39.1) ccw projected
  line L27 (68.5, 39.1) -> (68.5, 22.1) projected
  arc A33 (67.5, 21.1) -> (68.5, 22.1) centre (67.5, 22.1) ccw projected
  line L28 (67.5, 21.1) -> (35.5, 21.1) projected
  arc A34 (34.5, 22.1) -> (35.5, 21.1) centre (35.5, 22.1) ccw projected
  circle A35 centre (35.75, 43.95) radius 3 projected
  circle A36 centre (67.25, 43.95) radius 3 projected
  circle A37 centre (67.25, 14.25) radius 3 projected
  circle A38 centre (35.75, 14.25) radius 3 projected
  line L29 (-45, -48) -> (24, -48)
  line L30 (26, -50) -> (26, -54.5)
  line L31 (26, -54.5) -> (-47, -54.5)
  line L32 (-47, -54.5) -> (-47, -50)
  line L33 (26, -33.5) -> (26, -26.745) projected
  line L34 (-47, -26.745) -> (-47, -33.5) projected
  arc A39 (-45, -48) -> (-47, -50) centre (-45, -50) ccw
  arc A40 (26, -50) -> (24, -48) centre (24, -50) ccw
  arc A41 (-47, -33.5) -> (-45, -35.5) centre (-45, -33.5) ccw projected
  line L35 (-46.5, -50) -> (-46.5, -54)
  line L36 (-46.5, -54) -> (25.5, -54)
  line L37 (25.5, -54) -> (25.5, -50)
  arc A42 (25.5, -50) -> (24, -48.5) centre (24, -50) ccw
  line L38 (24, -48.5) -> (-45, -48.5)
  arc A43 (-45, -48.5) -> (-46.5, -50) centre (-45, -50) ccw
  line L39 (-46.5, -54) -> (-46.5, -54.5)
  line L40 (25.5, -54) -> (25.5, -54.5)
  point P0 (0, 0)
  point P1 (-47, -48)
  dimension "d113" = 6.5
  dimension "d115" = 0.5
  constraints: 20 end point, 8 point on circle, 4 centre point, 4 parallel, 4 point on line, 4 tangent, 2 collinear, 2 equal radius, 2 perpendicular, 1 horizontal, 5 other
  measures "d113" distance of L31.end point (-47, -48)
  measures "d115" distance between parallel lines of L35 L32
extrude "Extrusion9" add sketch "Sketch14" along normal up to surface (0.01 mm away) contours L29 A40 L30 L31 L40 L37 A42 L38 A43 L35 L39 L32 A39
sketch "Sketch16" plane through (0, 0, 1.6) normal (0, 0, 1) x (1, 0, 0)
  line L0 (16, -33.5) -> (16, -26.745) projected
  arc A0 (16, -14.255) -> (16, -26.745) centre (21, -20.5) ccw projected
  line L1 (16, -14.255) -> (16, -6) projected
  arc A1 (26, -6) -> (16, -6) centre (21, -6) ccw projected
  line L2 (26, -6) -> (26, -14.255) projected
  arc A2 (26, -26.745) -> (26, -14.255) centre (21, -20.5) ccw projected
  line L3 (26, -26.745) -> (26, -33.5) projected
  arc A3 (24, -35.5) -> (26, -33.5) centre (24, -33.5) ccw projected
  line L4 (24, -35.5) -> (18, -35.5) projected
  arc A4 (16, -33.5) -> (18, -35.5) centre (18, -33.5) ccw projected
  line L5 (-5, -33.5) -> (-5, -26.745) projected
  arc A5 (-5, -14.255) -> (-5, -26.745) centre (0, -20.5) ccw projected
  line L6 (-5, -14.255) -> (-5, -6) projected
  arc A6 (5, -6) -> (-5, -6) centre (0, -6) ccw projected
  line L7 (5, -6) -> (5, -14.255) projected
  arc A7 (5, -26.745) -> (5, -14.255) centre (0, -20.5) ccw projected
  line L8 (5, -26.745) -> (5, -33.5) projected
  arc A8 (3, -35.5) -> (5, -33.5) centre (3, -33.5) ccw projected
  line L9 (3, -35.5) -> (-3, -35.5) projected
  arc A9 (-5, -33.5) -> (-3, -35.5) centre (-3, -33.5) ccw projected
  line L10 (-26, -33.5) -> (-26, -26.745) projected
  arc A10 (-26, -14.255) -> (-26, -26.745) centre (-21, -20.5) ccw projected
  line L11 (-26, -14.255) -> (-26, -6) projected
  arc A11 (-16, -6) -> (-26, -6) centre (-21, -6) ccw projected
  line L12 (-16, -6) -> (-16, -14.255) projected
  arc A12 (-16, -26.745) -> (-16, -14.255) centre (-21, -20.5) ccw projected
  line L13 (-16, -26.745) -> (-16, -33.5) projected
  arc A13 (-18, -35.5) -> (-16, -33.5) centre (-18, -33.5) ccw projected
  line L14 (-18, -35.5) -> (-24, -35.5) projected
  arc A14 (-26, -33.5) -> (-24, -35.5) centre (-24, -33.5) ccw projected
  line L15 (-47, -33.5) -> (-47, -26.745) projected
  arc A15 (-47, -14.255) -> (-47, -26.745) centre (-42, -20.5) ccw projected
  line L16 (-47, -14.255) -> (-47, -6) projected
  arc A16 (-37, -6) -> (-47, -6) centre (-42, -6) ccw projected
  line L17 (-37, -6) -> (-37, -14.255) projected
  arc A17 (-37, -26.745) -> (-37, -14.255) centre (-42, -20.5) ccw projected
  line L18 (-37, -26.745) -> (-37, -33.5) projected
  arc A18 (-39, -35.5) -> (-37, -33.5) centre (-39, -33.5) ccw projected
  line L19 (-39, -35.5) -> (-45, -35.5) projected
  arc A19 (-47, -33.5) -> (-45, -35.5) centre (-45, -33.5) ccw projected
  circle A20 centre (10.5, -14) radius 3.5 projected
  circle A21 centre (-10.5, -14) radius 3.5 projected
  circle A22 centre (31.5, -14) radius 3.5 projected
  circle A23 centre (-31.5, -14) radius 3.5 projected
  circle A24 centre (35.75, 14.25) radius 3 projected
  circle A25 centre (67.25, 14.25) radius 3 projected
  circle A26 centre (67.25, 43.95) radius 3 projected
  circle A27 centre (35.75, 43.95) radius 3 projected
  line L20 (34.5, 22.1) -> (34.5, 39.1) projected
  arc A28 (35.5, 40.1) -> (34.5, 39.1) centre (35.5, 39.1) ccw projected
  line L21 (35.5, 40.1) -> (67.5, 40.1) projected
  arc A29 (68.5, 39.1) -> (67.5, 40.1) centre (67.5, 39.1) ccw projected
  line L22 (68.5, 39.1) -> (68.5, 22.1) projected
  arc A30 (67.5, 21.1) -> (68.5, 22.1) centre (67.5, 22.1) ccw projected
  line L23 (67.5, 21.1) -> (35.5, 21.1) projected
  arc A31 (34.5, 22.1) -> (35.5, 21.1) centre (35.5, 22.1) ccw projected
  circle A32 centre (-53.5, 13.5) radius 1.7 projected
  circle A33 centre (-58.5, 13.5) radius 1.7 projected
  circle A34 centre (-63.5, 13.5) radius 1.7 projected
  circle A35 centre (-68.5, 13.5) radius 1.7 projected
  circle A36 centre (63, -20.5) radius 8 projected
  line L24 (49, -24.373) -> (49, -33.5) projected
  arc A37 (47, -35.5) -> (49, -33.5) centre (47, -33.5) ccw projected
  line L25 (47, -35.5) -> (37, -35.5) projected
  arc A38 (35, -33.5) -> (37, -35.5) centre (37, -33.5) ccw projected
  line L26 (35, -33.5) -> (35, -24.373) projected
  arc A39 (37, -14.255) -> (35, -24.373) centre (42, -20.5) ccw projected
  line L27 (37, -14.255) -> (37, -6) projected
  arc A40 (47, -6) -> (37, -6) centre (42, -6) ccw projected
  line L28 (47, -6) -> (47, -14.255) projected
  arc A41 (49, -24.373) -> (47, -14.255) centre (42, -20.5) ccw projected
  circle A42 centre (-63, -20.5) radius 8 projected
  line L29 (-47, -54.5) -> (-47, -50) projected
  arc A43 (-45, -48) -> (-47, -50) centre (-45, -50) ccw projected
  line L30 (-45, -48) -> (24, -48) projected
  arc A44 (26, -50) -> (24, -48) centre (24, -50) ccw projected
  line L31 (26, -50) -> (26, -54.5) projected
  line L32 (26, -54.5) -> (63.4689, -54.5) projected
  arc A45 (63.4689, -54.5) -> (64.3647, -53.0556) centre (63.4689, -53.5) ccw projected
  arc A46 (69.0556, -48.3647) -> (64.3647, -53.0556) centre (67.5, -51.5) ccw projected
  arc A47 (69.0556, -48.3647) -> (70.5, -47.4689) centre (69.5, -47.4689) ccw projected
  line L33 (70.5, -47.4689) -> (70.5, -30.5) projected
  arc A48 (71.3276, -28.431) -> (70.5, -30.5) centre (73.5, -30.5) ccw projected
  arc A49 (71.3276, -28.431) -> (71.3276, -12.569) centre (63, -20.5) ccw projected
  arc A50 (70.5, -10.5) -> (71.3276, -12.569) centre (73.5, -10.5) ccw projected
  line L34 (70.5, -10.5) -> (70.5, 9.6199) projected
  arc A51 (71, 10.9428) -> (70.5, 9.6199) centre (72.5, 9.6199) ccw projected
  arc A52 (71, 10.9428) -> (72.25, 14.25) centre (67.25, 14.25) ccw projected
  line L35 (72.25, 14.25) -> (72.25, 43.95) projected
  arc A53 (72.25, 43.95) -> (71, 47.2572) centre (67.25, 43.95) ccw projected
  arc A54 (70.6186, 47.9015) -> (71, 47.2572) centre (72.5, 48.5801) ccw projected
  arc A55 (70.6186, 47.9015) -> (69.194, 48.4372) centre (69.678, 47.5622) ccw projected
  arc A56 (64.3647, 53.0556) -> (69.194, 48.4372) centre (67.5, 51.5) ccw projected
  arc A57 (64.3647, 53.0556) -> (63.4689, 54.5) centre (63.4689, 53.5) ccw projected
  line L36 (63.4689, 54.5) -> (-63.4689, 54.5) projected
  arc A58 (-63.4689, 54.5) -> (-64.3647, 53.0556) centre (-63.4689, 53.5) ccw projected
  arc A59 (-69.0556, 48.3647) -> (-64.3647, 53.0556) centre (-67.5, 51.5) ccw projected
  arc A60 (-69.0556, 48.3647) -> (-70.5, 47.4689) centre (-69.5, 47.4689) ccw projected
  line L37 (-70.5, 47.4689) -> (-70.5, 17.8589) projected
  arc A61 (-71.1087, 16.5323) -> (-70.5, 17.8589) centre (-72.25, 17.8589) ccw projected
  arc A62 (-71.1087, 16.5323) -> (-71.1087, 10.4677) centre (-68.5, 13.5) ccw projected
  arc A63 (-70.5, 9.1411) -> (-71.1087, 10.4677) centre (-72.25, 9.1411) ccw projected
  line L38 (-70.5, 9.1411) -> (-70.5, -10.5) projected
  arc A64 (-71.3276, -12.569) -> (-70.5, -10.5) centre (-73.5, -10.5) ccw projected
  arc A65 (-71.3276, -12.569) -> (-71.3276, -28.431) centre (-63, -20.5) ccw projected
  arc A66 (-70.5, -30.5) -> (-71.3276, -28.431) centre (-73.5, -30.5) ccw projected
  line L39 (-70.5, -30.5) -> (-70.5, -47.4689) projected
  arc A67 (-70.5, -47.4689) -> (-69.0556, -48.3647) centre (-69.5, -47.4689) ccw projected
  arc A68 (-64.3647, -53.0556) -> (-69.0556, -48.3647) centre (-67.5, -51.5) ccw projected
  arc A69 (-64.3647, -53.0556) -> (-63.4689, -54.5) centre (-63.4689, -53.5) ccw projected
  line L40 (-63.4689, -54.5) -> (-47, -54.5) projected
  circle A70 centre (63, -20.5) radius 11
  line L41 (56, -12.0147) -> (70, -12.0147)
  line L42 (70, -12.0147) -> (70, -6.5)
  line L43 (70, -6.5) -> (58, -6.5)
  line L44 (56, -8.5) -> (56, -12.0147)
  arc A71 (58, -6.5) -> (56, -8.5) centre (58, -8.5) ccw
  arc A72 (70, -10.5) -> (70.9655, -12.9138) centre (73.5, -10.5) ccw
  arc A73 (70.5, -10.5) -> (71.3276, -12.569) centre (73.5, -10.5) ccw projected
  arc A74 (55.0345, -12.9138) -> (56, -10.5) centre (52.5, -10.5) ccw
  point P0 (0, 0)
  dimension "d133" = 22
  dimension "d134" = 0.5
  dimension "d135" = 0.5
  dimension "d136" = 6
  dimension "d137" = 2
  constraints: 10 point on circle, 8 end point, 6 tangent, 4 centre point, 2 parallel, 2 point on line, 1 coincident, 1 concentric, 1 equal radius, 1 horizontal, 1 perpendicular
  measures "d133" diameter of A70
  measures "d134" radial gap between concentric circles of A49 A70
  measures "d135" distance between parallel lines of L34 L42
  measures "d136" distance edge to line of A36 L43
  measures "d137" radius of A71
extrude "Extrusion12" add sketch "Sketch16" along normal up to surface (0.01 mm away) contours A70 L41 | A70 L42 A72 | A74 L44 A70 | L41 A70 | A70 L44 A71 L43 L42
pattern_circular "Circular Pattern1" count 2 over 360 about axis through (0, -20.5, -179.4319) along (0, 0, 1) of "Extrusion12"
sketch "Sketch18" plane through (0, 0, 1.6) normal (0, 0, 1) x (1, 0, 0)
  circle A0 centre (-68.5, 13.5) radius 1.7 projected
  circle A1 centre (-53.5, 13.5) radius 1.7 projected
  line L0 (-68.5, 13.5) -> (-53.5, 13.5) construction
  line L1 (-68.5, 10) -> (-53.5, 10)
  line L2 (-53.5, 17) -> (-68.5, 17)
  arc A2 (-68.5, 17) -> (-68.5, 10) centre (-68.5, 13.5) ccw
  arc A3 (-53.5, 10) -> (-53.5, 17) centre (-53.5, 13.5) ccw
  arc A4 (-71.1087, 16.5323) -> (-71.1087, 10.4677) centre (-68.5, 13.5) ccw projected
  line L3 (-52, 5) -> (-70, 22) construction
  line L4 (-70, 5) -> (-52, 22) construction
  line L5 (-70.5, 17.8589) -> (-70.5, 47.4689) projected
  arc A5 (-70.7826, 16.1532) -> (-70, 17.8589) centre (-72.25, 17.8589) ccw
  arc A6 (-71.1087, 16.5323) -> (-70.5, 17.8589) centre (-72.25, 17.8589) ccw projected
  line L6 (-70, 17) -> (-52, 17)
  line L7 (-52, 17) -> (-52, 20)
  line L8 (-54, 22) -> (-70, 22)
  line L9 (-70, 22) -> (-70, 17)
  arc A7 (-52, 17.8589) -> (-51.2174, 16.1532) centre (-49.75, 17.8589) ccw
  arc A8 (-52, 20) -> (-54, 22) centre (-54, 20) ccw
  circle A9 centre (-63.5, 13.5) radius 1.7 projected
  circle A10 centre (-58.5, 13.5) radius 1.7 projected
  point P0 (0, 0)
  point P1 (-61, 13.5)
  point P2 (-62, 22)
  point P3 (-61, 17)
  dimension "d143" = 0.5
  dimension "d146" = 5
  dimension "d147" = 2
  constraints: 20 end point, 12 point on circle, 10 tangent, 5 centre point, 5 midpoint, 3 parallel, 2 horizontal, 2 point on line, 1 coincident, 1 collinear, 1 equal radius, 1 perpendicular, 1 vertical alignment
  measures "d143" radial gap between concentric circles of A2 A4
  measures "d146" distance between parallel lines of L2 L8
  measures "d147" radius of A8
extrude "Extrusion13" add sketch "Sketch18" along normal up to surface (0.005 mm away)
sketch "Sketch19" plane through (0, 0, 1.6) normal (0, 0, 1) x (1, 0, 0)
  line L0 (-105.2072, -40.5) -> (113.7805, -40.5) construction
  line L1 (113.7126, -1) -> (-91.0678, -1) construction
  line L2 (-67.5, -55.5) -> (67.5, -55.5) projected
  line L3 (-55.6132, -41.5) -> (-56.7679, -43.5)
  line L4 (-56.7679, -43.5) -> (-60.2321, -43.5)
  line L5 (-60.2321, -43.5) -> (-61.9641, -40.5)
  line L6 (-61.9641, -40.5) -> (-60.2321, -37.5)
  line L7 (-60.2321, -37.5) -> (-56.7679, -37.5)
  line L8 (-56.7679, -37.5) -> (-55.6132, -39.5)
  line L9 (-60.2321, -37.5) -> (-60.2321, -43.5)
  line L10 (-60.2321, -43.5) -> (-70.5, -43.5)
  line L11 (-70.5, -43.5) -> (-70.5, -37.5)
  line L12 (-70.5, -37.5) -> (-60.2321, -37.5)
  line L13 (-70.5, -47.4689) -> (-70.5, -30.5) projected
  line L14 (-60.2321, -43) -> (-57.0566, -43)
  line L15 (-57.0566, -43) -> (-56.0463, -41.25)
  line L16 (-56.0463, -39.75) -> (-57.0566, -38)
  line L17 (-57.0566, -38) -> (-60.2321, -38)
  line L18 (-60.2321, -38) -> (-70, -38)
  line L19 (-70, -38) -> (-70, -43)
  line L20 (-70, -43) -> (-60.2321, -43)
  line L21 (-70, -38) -> (-70, -43)
  line L22 (-70, -43) -> (-70.5, -43)
  line L23 (-70.5, -43) -> (-70.5, -38)
  line L24 (-70.5, -38) -> (-70, -38)
  arc A0 (-55.6132, -41.5) -> (-55.6132, -39.5) centre (-57.3453, -40.5) ccw
  arc A1 (-56.0463, -41.25) -> (-56.0463, -39.75) centre (-57.3453, -40.5) ccw
  line L25 (-60.5207, -38) -> (-60.2321, -38)
  line L26 (-60.5207, -43) -> (-60.2321, -43)
  line L27 (52.0359, -40.5) -> (53.7679, -37.5)
  line L28 (53.7679, -37.5) -> (57.2321, -37.5)
  line L29 (57.2321, -37.5) -> (58.5311, -39.75)
  line L30 (58.5311, -41.25) -> (57.2321, -43.5)
  line L31 (57.2321, -43.5) -> (53.7679, -43.5)
  line L32 (53.7679, -43.5) -> (52.0359, -40.5)
  line L33 (57.2321, -37.5) -> (57.2321, -43.5)
  line L34 (57.2321, -43.5) -> (70.5, -43.5)
  line L35 (70.5, -43.5) -> (70.5, -37.5)
  line L36 (70.5, -37.5) -> (57.2321, -37.5)
  line L37 (70.5, -30.5) -> (70.5, -47.4689) projected
  line L38 (58.0981, -38) -> (70, -38)
  line L39 (70, -38) -> (70, -43)
  line L40 (70, -43) -> (58.0981, -43)
  line L41 (58.0981, -38) -> (58.9641, -39.5)
  line L42 (58.9641, -41.5) -> (58.0981, -43)
  arc A2 (58.9641, -41.5) -> (58.9641, -39.5) centre (57.2321, -40.5) ccw
  arc A3 (58.5311, -41.25) -> (58.5311, -39.75) centre (57.2321, -40.5) ccw
  line L43 (70, -38) -> (70, -43)
  line L44 (70, -43) -> (70.5, -43)
  line L45 (70.5, -43) -> (70.5, -38)
  line L46 (70.5, -38) -> (70, -38)
  line L47 (-70.5, 3) -> (-57.8094, 3)
  line L48 (-57.8094, 3) -> (-57.8094, -5)
  line L49 (-57.8094, -5) -> (-70.5, -5)
  line L50 (-70.5, -5) -> (-70.5, 3)
  line L51 (-51.7472, -2.5) -> (-53.1906, -5)
  line L52 (-53.1906, -5) -> (-57.8094, -5)
  line L53 (-57.8094, -5) -> (-60.1188, -1)
  line L54 (-60.1188, -1) -> (-57.8094, 3)
  line L55 (-57.8094, 3) -> (-53.1906, 3)
  line L56 (-53.1906, 3) -> (-51.7472, 0.5)
  line L57 (-70.5, -10.5) -> (-70.5, 9.1411) projected
  arc A4 (-51.7472, -2.5) -> (-51.7472, 0.5) centre (-54.3453, -1) ccw
  line L58 (-56.2585, 2.5) -> (-70, 2.5)
  line L59 (-70, 2.5) -> (-70, -4.5)
  line L60 (-70, -4.5) -> (-58.4547, -4.5)
  line L61 (-60.1534, 2.5) -> (-53.4793, 2.5)
  line L62 (-53.4793, 2.5) -> (-52.1802, 0.25)
  arc A5 (-52.1802, -2.25) -> (-52.1802, 0.25) centre (-54.3453, -1) ccw
  line L63 (-52.1802, -2.25) -> (-53.4793, -4.5)
  line L64 (-53.4793, -4.5) -> (-59.9323, -4.5)
  line L65 (-70, 2.5) -> (-70.5, 2.5)
  line L66 (-70.5, 2.5) -> (-70.5, -4.5)
  line L67 (-70.5, -4.5) -> (-70, -4.5)
  line L68 (-70, -4.5) -> (-70, 2.5)
  point P0 (0, 0)
  point P1 (-58.5, -40.5)
  point P2 (-55.0359, -40.5)
  point P3 (55.5, -40.5)
  point P4 (58.9641, -40.5)
  point P5 (-55.5, -1)
  point P6 (-50.8812, -1)
  dimension "d150" = 15
  dimension "d151" = 54.5
  dimension "d152" = 6
  dimension "d153" = 12
  dimension "d154" = 0.5
  dimension "d155" = 2
  dimension "d159" = 15
  dimension "d160" = 0.5
  dimension "d161" = 0.5
  dimension "d162" = 2
  dimension "d164" = 15
  dimension "d165" = 8
  dimension "d166" = 3
  dimension "d167" = 0.5
  constraints: 131 end point, 21 point on line, 15 parallel, 12 point on circle, 10 tangent, 6 centre point, 6 collinear, 6 perpendicular, 4 horizontal, 3 vertical, 2 concentric, 53 other
  measures "d150" distance between parallel lines of L0 L2
  measures "d151" distance between parallel lines of L1 L2
  measures "d152" distance between parallel lines of L10 L12
  measures "d153" distance from line of point (-58.5, -40.5) L11
  measures "d154" distance between parallel lines of L18 L12
  measures "d155" radius of A0
  measures "d159" distance from line of point (55.5, -40.5) L35
  measures "d160" distance between parallel lines of L34 L40
  measures "d161" distance between parallel lines of L42 L30
  measures "d162" radius of A2
  measures "d164" distance from line of L50 point (-55.5, -1)
  measures "d165" distance between parallel lines of L49 L47
  measures "d166" radius of A4
  measures "d167" distance between parallel lines of L55 L61
extrude "Extrusion14" add sketch "Sketch19" along normal up to surface (0.01 mm away) contours L3 L4 L9 L14 L15 A1 L16 L17 L7 L8 A0 | L10 L11 L22 L20 L5 | L5 L20 L9 | L9 L18 L6 | L6 L18 L24 L11 L12 | L36 L35 L46 L38 L41 A2 L42 L40 L44 L34 L30 A3 L29 | L47 L54 L58 L65 L50 | L55 L56 A4 L51 L52 L48 L64 L63 A5 L62 L61 L58 | L48 L58 L54 | L67 L60 L64 L53 L49 L50 | L48 L53 L64